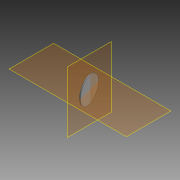
# Autodesk Inventor part: butterfly
Saved by Autodesk Inventor 2015 (Build 190159000, 159)
## iProperties
Created: 2015-09-04
Part Number: butterfly
Material: Brass, Soft Yellow
Description: insert part description/title
Document SubType Name: Modeling
Designer: francis
Density: 8.47 g/cm^3
Appearance: Brass - Satin
Author: francis
Part Category: insert part category here and press enter to fill value
Autodesk Inventor part; units mm, degrees
ref_plane "YZ Plane" through (0, 0, 0) normal (1, 0, 0) x (0, 1, 0)
ref_plane "XY Plane" through (0, 0, 0) normal (0, 0, 1) x (1, 0, 0)
ref_plane "Work Plane1" through (0, 0, 0) normal (0, 0, 1) x (1, 0, 0)
sketch "Sketch1" plane through (0, 0, 0) normal (0, 0, 1) x (1, 0, 0)
  line L0 (-120, -14) -> (-22.588, -14) construction
  line L1 (-120, 14) -> (-22.588, 14) construction
  line L2 (-58.0302, -14) -> (-60.5225, -14) construction
  line L3 (-56.6631, -13.7412) -> (-64.0963, 14)
  line L4 (-65.0622, 13.7412) -> (-57.629, -14)
  line L5 (-53.2531, -14) -> (-57.629, -14)
  line L6 (-60.345, 0) -> (-61.3803, 0) construction
  line L7 (-144, 0) -> (24, 0) construction
  line L8 (-60.8627, 54.7596) -> (-60.8627, -83.5575) construction
  line L9 (-60.8627, 20.7403) -> (-60.8627, -23.5336) construction
  line L10 (-47.8265, 0) -> (-82.556, 0) construction
  line L11 (-64.0963, 14) -> (-65.0622, 13.7412)
  line L12 (-57.629, -14) -> (-56.6631, -13.7412)
  point P0 (0, 0)
  point P1 (-60.8627, 0)
  dimension "d1" = 15
  dimension "d2" = 1
  constraints: 26 end point, 12 point on line, 3 horizontal, 2 midpoint, 2 perpendicular, 1 collinear, 1 parallel, 1 vertical, 8 other
  measures "d1" angle of L9 L4
  measures "d2" distance between parallel lines of L4 L3
extrude "Extrusion1" add sketch "Sketch1" along normal blind 30 and the other way blind 30
ref_plane "Work Plane2" through (-60.8627, 0, -16) normal (1, 0, 0) x (0, 0, -1)
sketch "Sketch2" plane through (-60.8627, 0, -16) normal (1, 0, 0) x (0, 0, -1)
  circle A0 centre (-16, 0) radius 14 projected
  point P0 (-16, 0)
extrude "Extrusion2" cut sketch "Sketch2" along normal mid plane 30 keep common part
ref_plane "Work Plane3" through (-57.1461, -13.8706, 2.6795) normal (0.9659258, 0.258819, 0) x (0, 0, -1)
sketch "Sketch4" plane through (-57.1461, -13.8706, 2.6795) normal (0.9659258, 0.258819, 0) x (0, 0, -1)
  line L0 (16.6795, 14.4939) -> (16.6795, 14.2259) construction
  line L1 (16.6795, 14.4939) -> (-11.3205, 14.4939) construction
  line L2 (-11.3205, 14.4939) -> (-11.3205, 14.2259) construction
  line L3 (2.24, 1.3335) -> (2.24, 27.5313) construction
  circle A0 centre (9.74, 14.4939) radius 1.5
  circle A1 centre (-5.26, 14.4939) radius 1.5
  point P0 (2.6795, -1.3925)
  dimension "d11" = 7.5
  dimension "d12" = 7.5
  dimension "d20" = 3
  dimension "d21" = 3
  constraints: 4 end point, 4 point on line, 2 centre point, 2 coincident, 1 horizontal, 1 vertical
  measures "d11" distance from line of L3 point (-5.26, 14.494)
  measures "d12" distance from line of point (9.74, 14.494) L3
  measures "d20" diameter of A1
  measures "d21" diameter of A0
extrude "Extrusion3" cut sketch "Sketch4" against normal blind 30 and the other way blind 15
body "Solid1"
